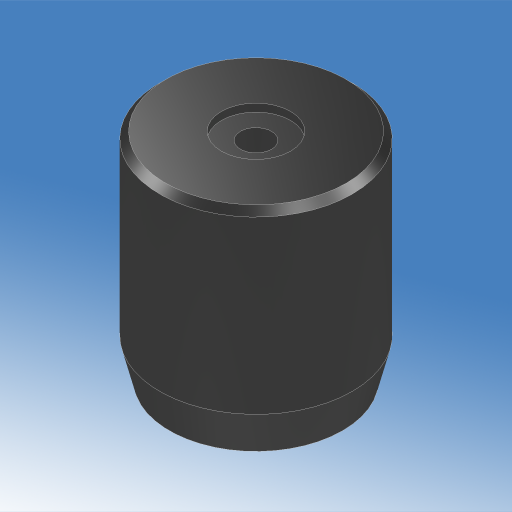
# Autodesk Inventor part: 5065
Saved by Autodesk Inventor 2024 (Build 280153000, 153)
## iProperties
Created: 2022-10-21
Part Number: 5065
Material: Generic
Document SubType Name: Modeling
Designer: kumpu
Density: 4.593 g/cm^3
Appearance: Glossy - Black
Mass: 476.272 g
Surface Area: 164.006 cm^2
Volume: 103.695 cm^3
Author: kumpu
Autodesk Inventor part; units mm, degrees
ref_plane "YZ Plane" through (0, 0, 0) normal (1, 0, 0) x (0, 1, 0)
ref_plane "XZ Plane" through (0, 0, 0) normal (0, 1, 0) x (-1, 0, 0)
ref_plane "XY Plane" through (0, 0, 0) normal (0, 0, 1) x (1, 0, 0)
sketch "Sketch1" plane through (0, 0, 0) normal (0, 0, 1) x (1, 0, 0)
  line L0 (4, 53.5) -> (4, 0)
  line L1 (4, 0) -> (24.75, 0)
  line L2 (24.75, 0) -> (24.75, 55.5)
  line L3 (24.75, 55.5) -> (0, 55.5)
  line L4 (24.75, 13) -> (24.75, 12)
  line L5 (24.75, 12) -> (15.6045, 12)
  line L6 (15.6045, 12) -> (15.6045, 13)
  line L7 (15.6045, 13) -> (24.75, 13)
  line L8 (24.75, 13) -> (24.75, 12)
  line L9 (4, 53.5) -> (8.87, 53.5)
  line L10 (8.87, 53.5) -> (8.87, 55.5)
  line L11 (0, 55.5) -> (0, 0)
  point P0 (8.87, 54.5)
  dimension "d2" = 55.5
  dimension "d32" = 1
  dimension "d33" = 12
  dimension "d36" = 2
  dimension "d37" = 49.5
  dimension "d38" = 8
  dimension "d39" = 17.74
  constraints: 24 end point, 5 perpendicular, 4 point on line, 2 horizontal, 2 parallel, 1 midpoint, 1 vertical
  measures "d2" distance of L1.end L2.end
  measures "d32" distance of L5.end L6.end
  measures "d33" distance between parallel lines of L1 L5
  measures "d36" distance of L9.end L10.end
  measures "d37" diameter of L2 L11
  measures "d38" diameter of L0 L11
  measures "d39" diameter of point (8.87, 54.5) L11
revolve "Revolution1" add sketch "Sketch1" angle 360 about axis through (0, 55.5, 0) along (0, -1, 0)
sketch "Sketch2" plane through (0, 0, 0) normal (0, -1, 0) x (1, 0, 0)
  circle A0 centre (19, 0) radius 2
  circle A1 centre (0, 0) radius 4 construction
  line L0 (0, 0) -> (19, 0) construction
  circle A2 centre (0, 19) radius 2
  circle A3 centre (-19, 0) radius 2
  circle A4 centre (0, -19) radius 2
  point P0 (0, 0)
  dimension "d5" = 4
  dimension "d6" = 19
  dimension "d9" = 360
  constraints: 4 centre point, 2 end point, 1 horizontal, 9 other
  measures "d5" diameter of A0
  measures "d6" distance of L0.start L0.end
extrude "Extrusion1" cut sketch "Sketch2" against normal blind 5
chamfer "Chamfer1" distance 1.6 angle 45 1 edges at (-24.75, 55.5, 0)
chamfer "Chamfer2" distance 2.5 distance2 10 1 edges at (-24.75, 0, 0) measured on face at (13.1279, 0, -6.9036)
body "Solid1"
